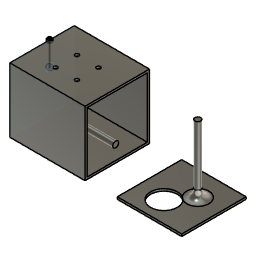
GearBox Box v17 (Autodesk Fusion 360 design; units mm, degrees)
Autodesk Fusion 360 part; units mm, degrees
note: some values were not read from the file. Chosen so that the rebuilt part matches the saved one: which bodies a step acts on.
sketch "Sketch1" plane through (0, 0, 0) normal (0, 0, 1) x (1, 0, 0)
  line L0 (35, -22.5) -> (-35, -22.5)
  line L1 (-35, -22.5) -> (-35, 22.5)
  line L2 (-35, 22.5) -> (35, 22.5)
  line L3 (35, 22.5) -> (35, -22.5)
  line L4 (35, -22.5) -> (-35, 22.5) construction
  line L5 (-35, -22.5) -> (35, 22.5) construction
  dimension "d1" = 70
  dimension "d2" = 45
  constraint horizontal L0
  constraint perpendicular L0 L1
  constraint parallel L0 L2
  constraint parallel L1 L3
  constraint coincident L4 origin
  constraint coincident L5 origin
  measures "d1" distance of L1.end L2.end
  measures "d2" distance of L0.end L1.end
extrude "Extrude1" add sketch "Sketch1" along normal blind 55 makes body 1
extrude "Extrude2" add 1 faces at (11.6667, -22.5, 18.3333) along direction (0, -1, 0) blind 15 on bodies 1 bodies 1
shell "Shell1" thickness 2 removed faces 1 at (35, 2.5, 18.3333) on bodies 1
extrude "Extrude3" add 1 faces at (-11.6667, 2.5, 0) along direction (0, 0, -1) blind 5 on bodies 1 bodies 1
extrude "Extrude4" cut 1 faces at (-10.3333, 1.8333, 2) along direction (0, 0, -1) blind 5 on bodies 1 bodies 1
sketch "Sketch2" plane through (-35, 0, 0) normal (-1, 0, 0) x (0, -1, 0)
  line L0 (37.5, -5) -> (37.5, 55)
  line L1 (37.5, 55) -> (-22.5, 55)
  line L2 (-22.5, 55) -> (-22.5, -5)
  line L3 (-22.5, -5) -> (37.5, -5)
  line L4 (-5, 55) -> (-5, 33) construction
  line L5 (-22.5, 33) -> (0.5, 33) construction
  dimension "d12" = 23
  constraint coincident L1 L4.start
  constraint perpendicular L1 L4
  constraint coincident L2 L5.start
  constraint perpendicular L4 L5
  measures "d12" distance of L5.start L5.end
sketch "Sketch3" plane through (-35, 0, 0) normal (-1, 0, 0) x (0, -1, 0)
  circle A0 centre (0.5, 33) radius 2.75
  dimension "d13" = 5.5
  measures "d13" diameter of A0
extrude "Extrude5" cut sketch "Sketch3" against normal blind 15 bodies 1
sketch "Sketch4" plane through (-35, 0, 0) normal (-1, 0, 0) x (0, -1, 0)
  line L0 (25, -5) -> (25, 19)
  line L1 (37.5, 19) -> (18.1, 19) construction
  dimension "d16" = 19.4
  constraint vertical L0
  constraint perpendicular L0 L1
  measures "d16" distance of L1.start L1.end
sketch "Sketch5" plane through (-35, 0, 0) normal (-1, 0, 0) x (0, -1, 0)
  circle A0 centre (18, 19) radius 2
  dimension "d17" = 4
  measures "d17" diameter of A0
extrude "Extrude6" cut sketch "Sketch5" against normal blind 31 bodies 1
extrude "Extrude7" add 1 faces at (-35, -10.7564, 2.3794) along direction (-1, 0, 0) blind 5 on bodies 1 bodies 1
sketch "Sketch6" plane through (0, -37.5, 0) normal (0, -1, 0) x (1, 0, 0)
  line L0 (35, -5) -> (35, 55)
  line L1 (35, 55) -> (-40, 55)
  line L2 (-40, 55) -> (-40, -5)
  line L3 (-40, -5) -> (35, -5)
  line L4 (-40, -5) -> (-35, -5) construction
  line L5 (-35, -5) -> (-38, -5)
  line L6 (-38, -5) -> (-38, 59.5786)
  line L7 (-38, 59.5786) -> (-35, 59.5786)
  line L8 (-35, 59.5786) -> (-35, -5)
  dimension "d22" = 3
  constraint coincident L2.end L3.start
  constraint coincident L3 L4.end
  constraint perpendicular L2 L4
  constraint horizontal L5
  constraint vertical L6
  constraint horizontal L7
  constraint vertical L8
  measures "d22" distance of L4.end L5.end
extrude "Extrude8" cut sketch "Sketch6" against normal blind 100 contours L1 L3 L5 L6 L8 bodies 1 makes body 2 at (-11.6667, 22.5, 35)
move_body "Move1" bodies 1 to x (0, 0, -1) y (0, 1, 0) z (1, 0, 0) at (70, 0, -45)
sketch "Sketch7" plane through (0, 0, -5) normal (0, 0, 1) x (-1, 0, 0)
  circle A0 centre (-89, 18) radius 2
  circle A1 centre (-103, 0.5) radius 2.75
  line L0 (-65, 37.5) -> (-125, 37.5)
  line L1 (-125, 37.5) -> (-125, -22.5)
  line L2 (-125, -22.5) -> (-65, -22.5)
  line L3 (-65, -22.5) -> (-65, 37.5)
  circle A2 centre (-89, 18) radius 11.5
  dimension "d25" = 23
  constraint concentric A0 A2
  measures "d25" diameter of A2
extrude "Extrude9" cut sketch "Sketch7" against normal blind 7 contours A2 bodies 1
extrude "Extrude10" add sketch "Sketch5" against normal blind 2 bodies 2
sketch "Sketch8" plane through (-35, 0, 0) normal (-1, 0, 0) x (0, -1, 0)
  line L0 (-22.5, 55) -> (-22.5, -5)
  line L1 (-22.5, -5) -> (37.5, -5)
  line L2 (37.5, -5) -> (37.5, 55)
  line L3 (37.5, 55) -> (-22.5, 55)
  circle A0 centre (0.5, 33) radius 2.75
  circle A1 centre (18, 19) radius 2.75
  dimension "d30" = 5.5
  measures "d30" diameter of A1
extrude "Extrude11" add sketch "Sketch8" against normal blind 74 contours A1 bodies 2
extrude "Extrude12" add 1 faces at (39, -17.6651, 19.5801) along direction (1, 0, 0) blind 5 on bodies 2 bodies 2
fillet "Fillet1" radius 4 1 edges at (-33, -15.4361, 18.0056) on bodies 2
move_body "Move2" bodies 1 to x (0, 0, 1) y (0, 1, 0) z (-1, 0, 0) at (58, 0, -72)
move_body "Move3" bodies 1 to x (1, 0, 0) y (0, 1, 0) z (0, 0, 1) at (0, 0, 2)
extrude "Extrude13" add sketch "Sketch3" against normal blind 100 bodies 1 2
extrude "Extrude14" cut sketch "Sketch3" against normal blind 20 bodies 1 makes body 3 at (65, 12.8226, 23.2865)
move_body "Move4" bodies 3 to x (0, 0, -1) y (0, 1, 0) z (1, 0, 0) at (70, 0, 60)
fillet "Fillet2" radius 7.5 1 edges at (103.9944, 2.0639, -3) on bodies 3
sketch "Sketch9" plane through (0, 0, -5) normal (0, 0, -1) x (1, 0, 0)
  circle A0 centre (89, 18) radius 11.5
  line L0 (65, -22.5) -> (125, -22.5)
  line L1 (125, -22.5) -> (125, 37.5)
  line L2 (125, 37.5) -> (65, 37.5)
  line L3 (65, 37.5) -> (65, -22.5)
  circle A1 centre (89, 18) radius 12.5
  dimension "d43" = 25
  constraint concentric A0 A1
  measures "d43" diameter of A1
extrude "Extrude15" cut sketch "Sketch9" against normal blind 20 contours A1 bodies 3
extrude "Extrude16" add 1 faces at (102.4836, -1.2574, 75) along direction (0, 0, 1) blind 5 on bodies 3 bodies 3
sketch "Sketch10" plane through (0, 0, 0) normal (0, 0, 1) x (1, 0, 0)
  line L0 (102.9, 0) -> (102.7, 0) construction
  constraint horizontal L0
extrude "Extrude17" cut 1 faces at (102.4836, -1.2574, 80) along direction (0, 0, -1) blind 10 on bodies 3 bodies 3
move_body "Move5" bodies 3 to x (0, 0, 1) y (0, 1, 0) z (-1, 0, 0) at (110, 0, -70)
extrude "Extrude18" cut 1 faces at (40, 0.4167, 34.247) along direction (1, 0, 0) blind 10 on bodies 3 bodies 3
sketch "Sketch11" plane through (-35, 0, 0) normal (-1, 0, 0) x (0, -1, 0)
  circle A0 centre (0.5, 33) radius 2.75
  line L0 (-22.5, 55) -> (-22.5, -5)
  line L1 (-22.5, -5) -> (37.5, -5)
  line L2 (37.5, -5) -> (37.5, 55)
  line L3 (37.5, 55) -> (-22.5, 55)
  line L4 (0.5, 33) -> (0.5, 55)
  constraint coincident A0.centre L4.start
  constraint coincident L3 L4.end
  constraint perpendicular L3 L4
extrude "Extrude19" add 1 faces at (-10.3333, 1.8333, 53) along direction (0, 0, -1) blind 5 on bodies 1 bodies 1
extrude "Extrude20" cut 1 faces at (-11.6667, 2.5, 55) along direction (0, 0, -1) blind 5 on bodies 1 bodies 1
extrude "Extrude21" add 1 faces at (-11.6667, 2.5, 50) along direction (0, 0, 1) blind 5 on bodies 1 bodies 1
extrude "Extrude22" cut 1 faces at (-10.3333, 1.8333, 48) along direction (0, 0, 1) blind 5 on bodies 1 bodies 1
sketch "Sketch12" plane through (0, 0, 55) normal (0, 0, 1) x (-1, 0, 0)
  line L0 (35, -22.5) -> (35, 37.5)
  line L1 (35, 37.5) -> (-35, 37.5)
  line L2 (-35, 37.5) -> (-35, -22.5)
  line L3 (-35, -22.5) -> (35, -22.5)
  circle A0 centre (-10, 20) radius 1.8
  circle A1 centre (10, 20) radius 1.8
  dimension "d60" = 3.6
  dimension "d61" = 3.6
  measures "d60" diameter of A0
  measures "d61" diameter of A1
extrude "Extrude23" cut sketch "Sketch12" against normal blind 2 contours A0 | A1 bodies 1
move_body "Move6" bodies 3 to x (0, 0, -1) y (0, 1, 0) z (1, 0, 0) at (70, 0, 110)
sketch "Sketch13" plane through (0, 0, 55) normal (0, 0, 1) x (-1, 0, 0)
  circle A0 centre (-10, 20) radius 1.8
  circle A1 centre (10, 20) radius 1.8
  line L0 (35, -22.5) -> (35, 37.5)
  line L1 (35, 37.5) -> (-35, 37.5)
  line L2 (-35, 37.5) -> (-35, -22.5)
  line L3 (-35, -22.5) -> (35, -22.5)
  circle A2 centre (10, 0) radius 1.8
  circle A3 centre (-10, 0) radius 1.8
  dimension "d64" = 3.6
  dimension "d65" = 3.6
  measures "d64" diameter of A2
  measures "d65" diameter of A3
extrude "Extrude24" cut sketch "Sketch13" against normal blind 9 contours A2 | A3 bodies 1
